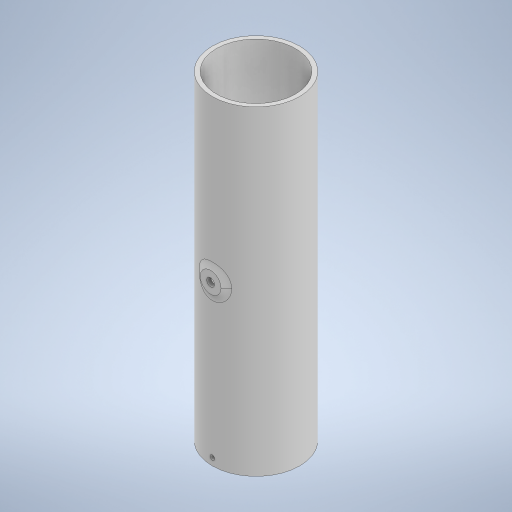
# Autodesk Inventor part: MotorTube
Saved by Autodesk Inventor 2023.2 (Build 272271030, 271C)
## iProperties
Created: 2023-03-06
Part Number: MotorTube
Material: Generic
Document SubType Name: Modeling
Designer: Lukas
Density: 1 g/cm^3
Appearance: Default
Author: Lukas
Autodesk Inventor part; units mm, degrees
ref_plane "YZ Plane" through (0, 0, 0) normal (1, 0, 0) x (0, 1, 0)
ref_plane "XZ Plane" through (0, 0, 0) normal (0, 1, 0) x (-1, 0, 0)
ref_plane "XY Plane" through (0, 0, 0) normal (0, 0, 1) x (1, 0, 0)
sketch "Motor Sketch" plane through (0, 0, 0) normal (0, 1, 0) x (-1, 0, 0)
  circle A0 centre (0, 0) radius 10.45
  circle A1 centre (0, 0) radius 9.45
  dimension "d0" = 20.9
  dimension "d3" = 18.9
  constraints: 2 centre point, 1 coincident, 1 concentric
  measures "d0" diameter of A0
  measures "d3" diameter of A1
extrude "Motor" add sketch "Motor Sketch" along normal mid plane 76.5
sketch "Zarazka Sketch" plane through (0, -38.25, 0) normal (0, -1, 0) x (1, 0, 0)
  circle A0 centre (0, 0) radius 9.45
  circle A1 centre (0, 0) radius 6.45
  dimension "d15" = 18.9
  dimension "d16" = 12.9
  constraints: 2 centre point, 2 coincident
  measures "d15" diameter of A0
  measures "d16" diameter of A1
extrude "Zarazka" add sketch "Zarazka Sketch" against normal blind 3.5
sketch "Sketch9" plane through (0, 0, 0) normal (0, 0, 1) x (1, 0, 0)
  line L0 (-1.1635, 1.9956) -> (1.1465, 2.0054)
  line L1 (1.1465, 2.0054) -> (2.31, 0.0098)
  line L2 (2.31, 0.0098) -> (1.1635, -1.9956)
  line L3 (1.1635, -1.9956) -> (-1.1465, -2.0054)
  line L4 (-1.1465, -2.0054) -> (-2.31, -0.0098)
  line L5 (-2.31, -0.0098) -> (-1.1635, 1.9956)
  point P0 (0, 0)
  point P1 (0, 0)
  dimension "d57" = 4.62
  constraints: 12 end point, 1 coincident, 13 other
  measures "d57" horizontal distance of L4.end L1.end
extrude "Motor Matice" cut sketch "Sketch9" along normal mid plane 19.7
sketch "Sketch10" plane through (0, 0, -9.85) normal (0, 0, 1) x (1, 0, 0)
  circle A0 centre (0, 0) radius 2.5
  dimension "d60" = 5
  constraints: 1 centre point, 1 coincident
  measures "d60" diameter of A0
extrude "Motor Lozisko Vyvisenina1" add sketch "Sketch10" against normal blind 1
sketch "Sketch11" plane through (0, 0, 9.85) normal (0, 0, -1) x (-1, 0, 0)
  circle A0 centre (0, 0) radius 2.5
  dimension "d63" = 5
  constraints: 1 centre point, 1 coincident
  measures "d63" diameter of A0
extrude "Motor Lozisko Vyvisenina2" add sketch "Sketch11" against normal blind 1
sketch "Sketch4" plane through (0, 0, 0) normal (0, 0, 1) x (1, 0, 0)
  point P0 (0, 0)
  point P1 (0, 0)
  constraints: 1 coincident
hole "TVC Inner Sroub1" at (0, 0, 0) direction (0, 0, -1) diameter 1.9 depth 20
sketch "Sketch5" plane through (0, 0, 0) normal (0, 0, 1) x (1, 0, 0)
  point P0 (0, 0)
  point P1 (0, 0)
  constraints: 1 coincident
hole "TVC Inner Sroub2" at (0, 0, 0) direction (0, 0, 1) diameter 1.9 depth 20
sketch "Sketch3" plane through (0, 0, 0) normal (0, 0, 1) x (1, 0, 0)
  line L0 (-10.45, -38.25) -> (10.45, -38.25) projected
  point P0 (0, 0)
  point P1 (0, -36.5)
  dimension "d73" = 1.75
  measures "d73" distance from line of L0 point (0, -36.5)
hole "Drzak1 Dira Tyc" [suppressed]
hole "Drzak2 Dira Tyc" at (0, -36.5, 0) direction (0, 0, 1) diameter 1.1 depth 20
sketch "Sketch12" plane through (0, 0, 0) normal (0, 0, 1) x (1, 0, 0)
  line L0 (-3, -33.4998) -> (3, -33.4998)
  line L1 (3, -33.4998) -> (3, -39.4998)
  line L2 (3, -39.4998) -> (-3, -39.4998)
  line L3 (-3, -39.4998) -> (-3, -33.4998)
  point P0 (0, 0)
  point P1 (0, -36.4998)
  dimension "d80" = 3
  dimension "d81" = 3
  dimension "d82" = 3
  dimension "d83" = 3
  constraints: 8 end point, 2 parallel, 1 horizontal, 1 perpendicular, 1 other
  measures "d80" distance from line of L2 point (0, -36.5)
  measures "d81" distance from line of point (0, -36.5) L0
  measures "d82" distance from line of point (0, -36.5) L3
  measures "d83" distance from line of L1 point (0, -36.5)
extrude "Motor Dira Tehlice" cut sketch "Sketch12" along normal blind 8.45
fillet "Motor Lozisko Vyvisenina Fillet" radius 3 2 edges at (-2.5, 0.0142, -10.1466) (2.5, 0.0142, 10.1466)
equation "\"d0\" = polomer_motor + tloustka_motor"
equation "\"d3\" = polomer_motor"
equation "\"d15\" = polomer_motor"
equation "\"d16\" = polomer_motor - zarazka"
equation "\"d19\" = zarazka_vyska"
equation "\"d57\" = m2_nut"
equation "\"d60\" = lozisko_inner"
equation "\"d63\" = lozisko_inner"
equation "\"d73\" = 0.5 * zarazka_vyska"
equation "\"d80\" = d82"
equation "\"d81\" = d82"
equation "\"d82\" = 0.5 * otvor_tehlice"
equation "\"d83\" = d82"
equation "\"d21\" = dira_tehlice"
equation "\"d66\" = dira_tehlice"
equation "\"tloustka_motor\" = 2"
equation "\"zarazka\" = 6"
equation "\"polomer_motor\" = 18.9"
equation "\"dira_tehlice\" = 1.1"
equation "\"m2_nut\" = 4.62"
equation "\"lozisko_inner\" = 5"
equation "\"zarazka_vyska\" = 3.5"
equation "\"otvor_tehlice\" = 6"
equation "\"d77\" = 0.5 * otvor_tehlice"
body "Solid1"
